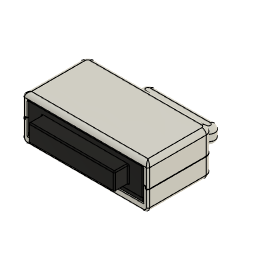
CBM8296_KB_Dongle v11 (Autodesk Fusion 360 design; units mm, degrees)
Autodesk Fusion 360 part; units mm, degrees
sketch "PCB" plane through (0, 0, 0) normal (0, 0, 1) x (1, 0, 0) in component "PCB"
  line L0 (53.0054, 0.0052) -> (53.0054, 25.0052)
  line L1 (53.0054, 25.0052) -> (0.0054, 25.0052)
  line L2 (0.0054, 25.0052) -> (0.0054, 0.0052)
  line L3 (0.0054, 0.0052) -> (53.0054, 0.0052)
  line L4 (46.9524, -0.1788) -> (47.9684, -0.1788)
  line L5 (46.4444, -6.1478) -> (46.4444, -0.6868)
  line L6 (45.9364, -6.6558) -> (7.0744, -6.6558)
  circle A0 centre (48.0054, 20.0052) radius 1.7463
  line L7 (47.9684, -0.1788) -> (51.9372, -0.1788)
  circle A1 centre (5.0054, 20.0052) radius 1.7463
  line L8 (5.4234, 15.3152) -> (5.3599, 15.3152)
  line L9 (52.7944, 2.1072) -> (47.6509, 2.1072)
  line L10 (46.4444, -0.6868) -> (46.9524, -0.1788)
  line L11 (45.9364, -6.4018) -> (45.9364, -0.6868)
  line L12 (52.7944, 0.2022) -> (0.2164, 0.2022)
  circle A2 centre (48.0054, 20.0052) radius 3.1789
  line L13 (0.2164, -0.1788) -> (1.0736, -0.1788)
  line L14 (5.3599, 2.1072) -> (0.2164, 2.1072)
  arc A3 (6.5664, -6.1478) -> (7.0744, -6.6558) centre (7.0744, -6.1478) ccw
  arc A4 (45.9364, -6.6558) -> (46.4444, -6.1478) centre (45.9364, -6.1478) ccw
  line L15 (5.0424, -6.5288) -> (5.0424, -0.0201)
  line L16 (1.0736, -0.1788) -> (6.0584, -0.1788)
  line L17 (0.2164, 0.2022) -> (0.2164, -0.1788)
  line L18 (0.2164, 0.2022) -> (0.2164, 2.1072)
  line L19 (51.9372, -0.1788) -> (52.7944, -0.1788)
  arc A5 (45.6824, -6.6558) -> (45.9364, -6.4018) centre (45.6824, -6.4018) ccw
  arc A6 (7.0744, -6.4018) -> (7.3284, -6.6558) centre (7.3284, -6.4018) ccw
  line L20 (52.7944, 13.7912) -> (52.7944, 2.1072)
  line L21 (7.0744, -6.4018) -> (7.0744, -0.6868)
  line L22 (47.6509, 15.3152) -> (5.4234, 15.3152)
  line L23 (5.3599, 7.6952) -> (5.3599, 2.1072)
  line L24 (47.6509, 7.6952) -> (47.6509, 2.1072)
  line L25 (1.0736, -0.1788) -> (1.0736, -6.5288)
  line L26 (0.2164, -0.1788) -> (52.7944, -0.1788)
  line L27 (47.9684, -6.5288) -> (47.9684, -0.1788)
  line L28 (5.4234, 15.3152) -> (1.6769, 15.3152)
  line L29 (47.6509, 7.6952) -> (47.6509, 15.3152)
  line L30 (47.6509, 7.6952) -> (5.3599, 7.6952)
  line L31 (52.7944, -0.1788) -> (52.7944, 0.2022)
  arc A7 (1.7404, 15.3152) -> (0.2164, 13.7277) centre (1.7404, 13.7899) ccw
  line L32 (51.9372, -6.5288) -> (47.9684, -6.5288)
  arc A8 (52.7944, 13.7912) -> (51.2704, 15.3152) centre (51.2704, 13.7912) ccw
  line L33 (5.3599, 7.6952) -> (5.3599, 15.3152)
  line L34 (1.0736, -6.5288) -> (5.0424, -6.5288)
  line L35 (52.7944, 0.2022) -> (0.2164, 0.2022)
  line L36 (51.9372, -0.1788) -> (51.9372, -6.5288)
  line L37 (47.6509, 15.3152) -> (51.2704, 15.3152)
  circle A9 centre (5.0054, 20.0052) radius 3.1789
  line L38 (52.7944, 0.2022) -> (52.7944, -0.1788)
  line L39 (52.7944, 2.1072) -> (52.7944, 0.2022)
  line L40 (6.5664, -0.6868) -> (6.5664, -6.1478)
  line L41 (0.2164, 2.1072) -> (0.2164, 13.7277)
  line L42 (6.0584, -0.1788) -> (46.9524, -0.1788)
  line L43 (0.2164, -0.1788) -> (0.2164, 0.2022)
  line L44 (47.6509, 2.1072) -> (5.3599, 2.1072)
  line L45 (6.0584, -0.1788) -> (6.5664, -0.6868)
  circle A10 centre (2.9854, 11.5052) radius 1.8034
  circle A11 centre (50.0254, 11.5052) radius 1.8034
extrude "Extrude1" add sketch "PCB" against normal blind 1.6 contours L0 L1 L2 L3 L8 L17 L18 L20 L22 L28 L31 A7 A8 L37 L38 L39 L41 L43 | L3 L12 L17 L31 L35 L38 L43 | L9 L12 L14 L18 L35 L39 L44 | L9 L20 L24 L29 A8 L37 | L14 L23 L28 A7 L33 L41 | L23 L24 L30 L44 | L8 L22 L28 L29 L30 L33 | A2 | A9 | A10 | A11 makes body 1 in component "PCB"
extrude "Extrude12" add sketch "PCB" along normal blind 10.2 contours L23 L24 L30 L44 | L8 L22 L28 L29 L30 L33 bodies 1 in component "PCB"
extrude "Extrude13" add sketch "PCB" along normal blind 12.5 contours L3 L4 L7 L13 L16 L17 L19 L26 L31 L38 L42 L43 | L3 L12 L17 L31 L35 L38 L43 | L9 L12 L14 L18 L35 L39 L44 bodies 1 in component "PCB"
extrude "Extrude14" add sketch "PCB" along normal blind 2.8 contours L9 L20 L24 L29 A8 L37 | L14 L23 L28 A7 L33 L41 bodies 1 in component "PCB"
extrude "Extrude15" add sketch "PCB" along normal blind 8.2 from surface at 2.15 contours L5 L6 L10 A3 A4 L26 L40 L42 L45 bodies 1 in component "PCB"
fillet "Fillet1" radius 0.508 14 edges at (6.5664, -3.4173, 10.35) (6.7152, -6.507, 10.35) (26.5054, -6.6558, 10.35) (46.2956, -6.507, 10.35) (46.4444, -3.4173, 10.35) (6.3124, -0.4328, 10.35) (6.5664, -3.4173, 2.15) (6.7152, -6.507, 2.15) (26.5054, -6.6558, 2.15) (46.2956, -6.507, 2.15) (46.4444, -3.4173, 2.15) (6.3124, -0.4328, 2.15) (46.6984, -0.4328, 10.35) (46.6984, -0.4328, 2.15) on bodies 1 in component "PCB"
ref_plane "WorkPlane1" through (0, 0, -3.1) normal (0, 0, 1) x (1, 0, 0) in component "bottom_shell"
sketch "bottom" plane through (0, 0, -3.1) normal (0, 0, 1) x (1, 0, 0) in component "bottom_shell"
  circle A0 centre (48.0054, 20.0052) radius 1.75
  circle A1 centre (5.0054, 20.0052) radius 1.75
  line L0 (52.5054, 29.8522) -> (0.5054, 29.8522)
  circle A2 centre (48.0054, 20.0052) radius 4.25
  circle A3 centre (5.0054, 20.0052) radius 4.25
  circle A4 centre (48.0054, 20.0052) radius 3
  circle A5 centre (5.0054, 20.0052) radius 3
  line L1 (40.5054, 34.8522) -> (40.5054, 39.8522) construction
  line L2 (40.5054, 39.8522) -> (12.5054, 39.8522) construction
  line L3 (40.5054, 39.8522) -> (40.5054, 39.501) construction
  arc A6 (40.5054, 39.8522) -> (40.5054, 45.8522) centre (40.5054, 42.8522) ccw
  arc A7 (40.5054, 39.8522) -> (40.5054, 29.8522) centre (40.5054, 34.8522) ccw
  line L4 (53.0054, 25.0052) -> (0.0054, 25.0052) construction
  line L5 (53.0054, 0.0052) -> (53.0054, 25.0052) construction
  line L6 (0.0054, 0.0052) -> (53.0054, 0.0052) construction
  line L7 (0.0054, 25.0052) -> (0.0054, 0.0052) construction
  circle A8 centre (5.0054, 20.0052) radius 1.7463 construction
  circle A9 centre (48.0054, 20.0052) radius 1.7463 construction
  line L8 (26.5054, 0.0052) -> (26.5054, 43) construction
  arc A10 (12.5054, 45.8522) -> (12.5054, 39.8522) centre (12.5054, 42.8522) ccw
  arc A11 (12.5054, 29.8522) -> (12.5054, 39.8522) centre (12.5054, 34.8522) ccw
  line L9 (12.5054, 45.8522) -> (40.5054, 45.8522)
  line L10 (-2.4946, 26.8522) -> (-2.4946, -0.1478)
  line L11 (-2.4946, -0.1478) -> (55.5054, -0.1478)
  line L12 (55.5054, -0.1478) -> (55.5054, 26.8522)
  arc A12 (55.5054, 26.8522) -> (52.5054, 29.8522) centre (52.5054, 26.8522) ccw
  arc A13 (0.5054, 29.8522) -> (-2.4946, 26.8522) centre (0.5054, 26.8522) ccw
  line L13 (-0.4946, 26.8522) -> (-0.4946, 1.8522)
  line L14 (-0.4946, 1.8522) -> (53.5054, 1.8522)
  line L15 (53.5054, 1.8522) -> (53.5054, 26.8522)
  arc A14 (53.5054, 26.8522) -> (52.5054, 27.8522) centre (52.5054, 26.8522) ccw
  line L16 (52.5054, 27.8522) -> (0.5054, 27.8522)
  arc A15 (0.5054, 27.8522) -> (-0.4946, 26.8522) centre (0.5054, 26.8522) ccw
  line L17 (-0.4946, 1.8522) -> (-0.4946, -0.1478)
  line L18 (53.5054, 1.8522) -> (53.5054, -0.1478)
  line L19 (54.3054, -0.1478) -> (54.3054, 26.8522)
  arc A16 (54.3054, 26.8522) -> (52.5054, 28.6522) centre (52.5054, 26.8522) ccw
  line L20 (52.5054, 28.6522) -> (0.5054, 28.6522)
  arc A17 (0.5054, 28.6522) -> (-1.2946, 26.8522) centre (0.5054, 26.8522) ccw
  line L21 (-1.2946, 26.8522) -> (-1.2946, -0.1478)
  circle A18 centre (2.9854, 11.5052) radius 1.8034 construction
  circle A19 centre (50.0254, 11.5052) radius 1.8034 construction
  circle A20 centre (2.9854, 11.5052) radius 2.75
  circle A21 centre (50.0254, 11.5052) radius 2.75
  line L22 (2.9854, 8.7552) -> (50.0254, 8.7552)
  line L23 (2.9854, 14.2552) -> (50.0254, 14.2552)
  point P0 (-2.4946, 29.8522)
  dimension "d181" = 3.5
  dimension "d182" = 3.5
  dimension "d190" = 8.5
  dimension "d191" = 8.5
  dimension "d194" = 6
  dimension "d195" = 6
  dimension "d236" = 10
  dimension "d238" = 5
  dimension "d239" = 6
  dimension "d265" = 14
  dimension "d267" = 30
  dimension "d268" = 58
  dimension "d269" = 3
  dimension "d271" = -1.2
  dimension "d288" = 5.5
  dimension "d289" = 5.5
  constraint coincident L1.start A7.centre
  constraint vertical L1
  constraint tangent L2 A6
  constraint perpendicular L2 L3
  constraint coincident A6.centre L3
  constraint coincident L3 A6.end
  constraint coincident L0 A7.end
  constraint coincident L6 L8.start
  constraint perpendicular L4 L8
  constraint symmetric L5 L7 L8
  constraint concentric A2 A9
  constraint concentric A4 A9
  constraint concentric A0 A9
  constraint concentric A3 A8
  constraint concentric A5 A8
  constraint concentric A1 A8
  constraint symmetric L1.end L8 L2.end
  constraint symmetric A6.end L8 A10.start
  constraint symmetric A6 L8 A10
  constraint symmetric A7.end L8 A11.start
  constraint symmetric A7 L8 A11
  constraint tangent A6 L9
  constraint perpendicular L0 L10
  constraint perpendicular L5 L11
  constraint perpendicular L0 L12
  constraint symmetric L8 L10 L12
  constraint tangent L0 A12
  constraint tangent L12 A12
  constraint coincident L0 P0
  constraint coincident P0 L10
  constraint tangent L0 A13
  constraint tangent L10 A13
  constraint equal A12 A13
  constraint coincident L11 L17.end
  constraint perpendicular L11 L17
  constraint coincident L11 L18.end
  constraint perpendicular L11 L18
  constraint concentric A18 A20
  constraint concentric A19 A21
  constraint horizontal L22
  constraint tangent A20 L22
  constraint tangent A21 L23
  constraint tangent A20 L23
  constraint coincident A20 L23.start
  constraint coincident A20 L22.start
  constraint coincident A21 L23.end
  constraint coincident A21 L22.end
  measures "d181" diameter of A0
  measures "d182" diameter of A1
  measures "d190" diameter of A2
  measures "d191" diameter of A3
  measures "d194" diameter of A4
  measures "d195" diameter of A5
  measures "d236" diameter of A7
  measures "d238" distance of L0 L1.start
  measures "d239" diameter of A6
  measures "d265" distance of L1.start L8
  measures "d267" distance of P0 L10.end
  measures "d268" distance of L10 L12
  measures "d269" radius of A12
  measures "d288" diameter of A20
  measures "d289" diameter of A21
extrude "Extrude1'" add sketch "bottom" against normal blind 2 separate body contours L0 L10 L11 L12 A12 A13 L19 A16 L20 A17 L21 | L0 A6 A7 A10 A11 L9 | L11 L13 L15 A14 L16 A15 L17 L18 L19 A16 L20 A17 L21 | L11 L14 L17 L18 | L13 L14 L15 A14 L16 A15 | A2 | A3 | A20 | A20 A21 L22 L23 | A21 makes body 2 in component "bottom_shell"
extrude "Extrude2" add sketch "bottom" along normal blind 1.5 contours A2 | A3 | A4 | A5 bodies 2 in component "bottom_shell"
extrude "Extrude3" add sketch "bottom" along normal blind 1 contours L11 L14 L17 L18 bodies 2 in component "bottom_shell"
extrude "Extrude4" add sketch "bottom" along normal blind 8.4 contours L11 L13 L15 A14 L16 A15 L17 L18 L19 A16 L20 A17 L21 bodies 2 in component "bottom_shell"
extrude "Extrude5" add sketch "bottom" along normal blind 7.4 contours L0 L10 L11 L12 A12 A13 L19 A16 L20 A17 L21 bodies 2 in component "bottom_shell"
extrude "Extrude6" add sketch "bottom" along normal blind 5 contours L0 A6 A7 A10 A11 L9 bodies 2 in component "bottom_shell"
fillet "Fillet8" radius 0.5 6 edges at (53.5054, 14.3522, -3.1) (53.2125, 27.5593, -3.1) (26.5054, 27.8522, -3.1) (-0.2017, 27.5593, -3.1) (-0.4946, 14.3522, -3.1) (26.5054, 1.8522, -3.1) on bodies 2 in component "bottom_shell"
fillet "Fillet9" radius 0.5 2 edges at (1.043, 21.5421, -3.1) (44.043, 21.5421, -3.1) on bodies 2 in component "bottom_shell"
chamfer "Chamfer2" distance 0.8 angle 45 2 edges at (1.043, 18.4683, -1.6) (44.043, 18.4683, -1.6) on bodies 2 in component "bottom_shell"
fillet "Fillet5" radius 2 16 edges at (46.5054, 29.8522, -5.1) (54.6267, 28.9735, -5.1) (55.5054, 13.3522, -5.1) (35.5054, 34.8522, -5.1) (43.5054, 42.8522, -5.1) (26.5054, 45.8522, -5.1) (9.5054, 42.8522, -5.1) (17.5054, 34.8522, -5.1) (6.5054, 29.8522, -5.1) (-1.6159, 28.9735, -5.1) (-2.4946, 13.3522, -5.1) (35.5054, 34.8522, 1.9) (43.5054, 42.8522, 1.9) (26.5054, 45.8522, 1.9) (9.5054, 42.8522, 1.9) (17.5054, 34.8522, 1.9) on bodies 2 in component "bottom_shell"
fillet "Fillet10" radius 0.75 5 edges at (55.5054, -0.1478, 0.6) (54.9196, -0.1478, -4.5142) (26.5054, -0.1478, -5.1) (-1.9088, -0.1478, -4.5142) (-2.4946, -0.1478, 0.6) on bodies 2 in component "bottom_shell"
ref_plane "WorkPlane1" through (0, 0, 13) normal (0, 0, 1) x (1, 0, 0) in component "top_shell"
sketch "top" plane through (0, 0, 13) normal (0, 0, 1) x (1, 0, 0) in component "top_shell"
  line L0 (52.5054, 29.8522) -> (0.5054, 29.8522)
  circle A0 centre (5.0054, 20.0052) radius 1.75 construction
  circle A1 centre (48.0054, 20.0052) radius 1.75 construction
  circle A2 centre (5.0054, 20.0052) radius 1.25
  circle A3 centre (48.0054, 20.0052) radius 1.25
  circle A4 centre (5.0054, 20.0052) radius 3.5
  circle A5 centre (48.0054, 20.0052) radius 3.5
  line L1 (-2.4946, 26.8522) -> (-2.4946, -0.1478)
  arc A6 (0.5054, 29.8522) -> (-2.4946, 26.8522) centre (0.5054, 26.8522) ccw
  arc A7 (55.5054, 26.8522) -> (52.5054, 29.8522) centre (52.5054, 26.8522) ccw
  line L2 (55.5054, -0.1478) -> (55.5054, 26.8522)
  line L3 (-2.4946, -0.1478) -> (55.5054, -0.1478)
  line L4 (53.5054, 1.8522) -> (53.5054, 26.8522)
  line L5 (53.5054, 1.8522) -> (53.5054, -0.1478)
  arc A8 (53.5054, 26.8522) -> (52.5054, 27.8522) centre (52.5054, 26.8522) ccw
  line L6 (52.5054, 27.8522) -> (0.5054, 27.8522)
  arc A9 (0.5054, 27.8522) -> (-0.4946, 26.8522) centre (0.5054, 26.8522) ccw
  line L7 (-0.4946, 26.8522) -> (-0.4946, 1.8522)
  line L8 (-0.4946, 1.8522) -> (-0.4946, -0.1478)
  line L9 (54.7054, -0.1478) -> (54.7054, 26.8522)
  arc A10 (54.7054, 26.8522) -> (52.5054, 29.0522) centre (52.5054, 26.8522) ccw
  line L10 (52.5054, 29.0522) -> (0.5054, 29.0522)
  arc A11 (0.5054, 29.0522) -> (-1.6946, 26.8522) centre (0.5054, 26.8522) ccw
  line L11 (-1.6946, 26.8522) -> (-1.6946, -0.1478)
  dimension "d213" = 2.5
  dimension "d214" = 2.5
  dimension "d220" = 7
  dimension "d221" = 7
  dimension "d281" = -0.8
  constraint concentric A0 A2
  constraint concentric A1 A3
  constraint concentric A2 A4
  constraint concentric A3 A5
  measures "d213" diameter of A2
  measures "d214" diameter of A3
  measures "d220" diameter of A4
  measures "d221" diameter of A5
extrude "Extrude1''" add sketch "top" along normal blind 2 separate body contours L0 L1 A6 A7 L2 L3 L9 A10 L10 A11 L11 | L3 L4 L5 A8 L6 A9 L7 L8 L9 A10 L10 A11 L11 | L3 L4 L5 A8 L6 A9 L7 L8 | A2 | A3 | A4 | A5 makes body 3 in component "top_shell"
extrude "Extrude2'" add sketch "top" against normal blind 12.8 contours A4 | A5 bodies 3 in component "top_shell"
extrude "Extrude3'" add sketch "top" against normal blind 7.5 contours L3 L4 L5 A8 L6 A9 L7 L8 L9 A10 L10 A11 L11 bodies 3 in component "top_shell"
extrude "Extrude4'" add sketch "top" against normal blind 8.5 contours L0 L1 A6 A7 L2 L3 L9 A10 L10 A11 L11 bodies 3 in component "top_shell"
extrude "Extrude5'" add sketch "top" against normal blind 8.5 contours L0 L1 A6 A7 L2 L3 L9 A10 L10 A11 L11 bodies 3 in component "top_shell"
fillet "Fillet1'" radius 1 2 edges at (1.7423, 18.7395, 13) (44.7423, 18.7395, 13) on bodies 3 in component "top_shell"
fillet "Fillet3" radius 1 5 edges at (-0.4946, 13.3522, 13) (-0.2017, 27.5593, 13) (26.5054, 27.8522, 13) (53.2125, 27.5593, 13) (53.5054, 13.3522, 13) on bodies 3 in component "top_shell"
fillet "Fillet4" radius 0.75 2 edges at (55.5054, -0.1478, 9.75) (-2.4946, -0.1478, 9.75) on bodies 3 in component "top_shell"
fillet "Fillet5'" radius 2 8 edges at (26.5054, 29.8522, 15) (-1.6159, 28.9735, 15) (-2.4946, 13.7272, 15) (-2.2749, 0.0719, 15) (26.5054, -0.1478, 15) (55.2857, 0.0719, 15) (55.5054, 13.7272, 15) (54.6267, 28.9735, 15) on bodies 3 in component "top_shell"
extrude "Extrude7" cut sketch "bottom" against normal blind 1 contours A20 | A20 A21 L22 L23 | A21 bodies 2 in component "bottom_shell"
fillet "Fillet11" radius 0.5 4 edges at (26.5054, 8.7552, -4.1) (0.2354, 11.5052, -4.1) (26.5054, 14.2552, -4.1) (52.7754, 11.5052, -4.1) on bodies 2 in component "bottom_shell"
component "PCB" placed x (1, 0, 0) y (0, 1, 0) z (0, 0, 1) at (0, 0, 0)
component "bottom_shell" placed x (1, 0, 0) y (0, 1, 0) z (0, 0, 1) at (0, 0, 0)
component "top_shell" placed x (1, 0, 0) y (0, 1, 0) z (0, 0, 1) at (0, 0, 0)
equation "pcb_thickness = 1.6 mm"
equation "below = 1.5 mm + pcb_thickness"
equation "wall = 2 mm"
equation "width = pcb_width + 1 mm + 2 * wall"
equation "length = pcb_length + r_corner + wall"
equation "above = 13 mm"
equation "pcb_width = 53 mm"
equation "pcb_length = 25 mm"
equation "r_corner = 3 mm"
equation "drill = 3.5 mm"
equation "d_screw = 7 mm"
equation "tol_x = 0.3 mm"
equation "tol_connector = 0.6 mm"
equation "d_post = 8.5 mm"
equation "d_post2 = 8 mm"
equation "bottom_height = 4.3 mm + below"
equation "overlap = 1 mm"
equation "top_height = above + below - bottom_height - tol_y"
equation "d35 = tol_connector"
equation "d37 = d35"
equation "tol_y = 0.2 mm"
equation "d154 = -pcb_thickness"
equation "d180 = -below"
equation "d181 = drill"
equation "d182 = drill"
equation "d190 = d_post"
equation "d191 = d_post"
equation "d195 = d194"
equation "d198 = -wall"
equation "d200 = below - pcb_thickness"
equation "d202 = below - pcb_thickness - 0.5 mm"
equation "d204 = bottom_height + overlap"
equation "d206 = bottom_height"
equation "d212 = above"
equation "d220 = d_screw"
equation "d221 = d_screw"
equation "d224 = wall"
equation "d226 = -above + tol_y"
equation "d228 = -top_height + overlap"
equation "d230 = -top_height"
equation "d232 = -top_height"
equation "d238 = d236 / 2"
equation "d267 = length"
equation "d268 = width"
equation "d269 = r_corner"
equation "d270 = -wall"
equation "d271 = -0.6 * wall"
equation "d281 = -0.4 * wall"
equation "d289 = d288"
equation "d290 = -wall / 2"
named bodies: "PCB", "top"
